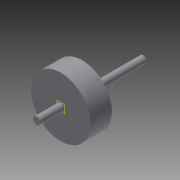
# Autodesk Inventor part: can
Saved by Autodesk Inventor 2013 (Build 170138000, 138)
## iProperties
Created: 2013-01-16
Part Number: can
Material: Generic
Document SubType Name: Modeling
Designer: geohot
Density: 1 g/cm^3
Author: geohot
Autodesk Inventor part; units mm, degrees
ref_plane "YZ Plane" through (0, 0, 0) normal (1, 0, 0) x (0, 1, 0)
ref_plane "XZ Plane" through (0, 0, 0) normal (0, 1, 0) x (-1, 0, 0)
ref_plane "XY Plane" through (0, 0, 0) normal (0, 0, 1) x (1, 0, 0)
sketch "Sketch1" plane through (0, 0, 0) normal (0, 0, 1) x (1, 0, 0)
  circle A0 centre (0, 0) radius 1.4605
  dimension "d0" = 2.921
  constraints: 1 centre point, 1 coincident
  measures "d0" diameter of A0
extrude "Extrusion1" add sketch "Sketch1" along normal blind 42.75
ref_plane "Work Plane1" through (0, 0, 33.14) normal (0, 0, 1) x (1, 0, 0)
sketch "Sketch2" plane through (0, 0, 33.14) normal (0, 0, 1) x (1, 0, 0)
  circle A0 centre (0, 0) radius 11.938
  dimension "d5" = 23.876
  constraints: 1 centre point, 1 coincident
  measures "d5" diameter of A0
extrude "Extrusion2" add sketch "Sketch2" against normal blind 8.636
sketch "Sketch3" plane through (0, 0, 24.504) normal (0, 0, -1) x (-1, 0, 0)
  circle A0 centre (0, 0) radius 1.4605 projected
  circle A1 centre (0, 0) radius 10.795
  dimension "d9" = 21.59
  constraints: 1 centre point, 1 coincident
  measures "d9" diameter of A1
extrude "Extrusion3" cut sketch "Sketch3" against normal blind 7.62
body "Solid1"
